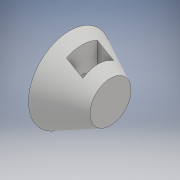
# Autodesk Inventor part: stollen_m4_vierkant
Saved by Autodesk Inventor 2018 (Build 220112000, 112)
## iProperties
Created: 2018-05-14
Part Number: stollen_m4_vierkant
Material: Generic
Document SubType Name: Modeling
Designer: bitbots
Density: 1 g/cm^3
Appearance: Default
Author: bitbots
Autodesk Inventor part; units mm, degrees
ref_plane "XZ Plane" through (0, 0, 0) normal (0, 1, 0) x (-1, 0, 0)
ref_plane "XY Plane" through (0, 0, 0) normal (0, 0, 1) x (1, 0, 0)
ref_plane "Work Plane1" through (7, 0, 0) normal (1, 0, 0) x (0, 1, 0)
sketch "Sketch1" plane through (0, 0, 0) normal (0, 1, 0) x (-1, 0, 0)
  line L0 (0, 0) -> (-10, 0)
  line L1 (0, 0) -> (0, -10)
  line L2 (-10, 0) -> (-10, -5)
  line L3 (-10, -5) -> (0, -10)
  dimension "d0" = 10
  dimension "d1" = 10
  dimension "d2" = 5
  constraints: 8 end point, 2 vertical, 1 horizontal
  measures "d0" distance of L0.start L0.end
  measures "d1" distance of L0.start L1.end
  measures "d2" distance of L0.end L2.end
revolve "Revolution1" add sketch "Sketch1" angle 360 about axis through (0, 0, 0) along (1, 0, 0)
sketch "Sketch2" plane through (7, 0, 0) normal (1, 0, 0) x (0, 1, 0)
  circle A0 centre (0, 0) radius 2.25
  dimension "d5" = 4.5
  constraints: 1 centre point, 1 coincident
  measures "d5" diameter of A0
extrude "Extrusion1" cut sketch "Sketch2" along normal blind 2 and the other way blind 10
sketch "Sketch3" plane through (7, 0, 0) normal (1, 0, 0) x (0, 1, 0)
  line L0 (0, 0) -> (3.75, 0)
  line L1 (3.75, -2.1651) -> (0, -4.3301)
  line L2 (0, -4.3301) -> (-3.75, -2.1651)
  line L3 (-3.75, -2.1651) -> (-3.75, 2.1651)
  line L4 (-3.75, 2.1651) -> (0, 4.3301)
  line L5 (0, 4.3301) -> (3.75, 2.1651)
  line L6 (3.75, 2.1651) -> (3.75, -2.1651)
  line L7 (-3.75, 14.6203) -> (-3.75, 2.1651)
  line L8 (-3.75, 14.6203) -> (3.75, 14.6203)
  line L9 (3.75, 14.6203) -> (3.75, 1.2022)
  line L10 (3.75, 1.2022) -> (-3.75, 1.2022)
  line L11 (-3.75, 1.2022) -> (-3.75, 14.6203)
  dimension "d15" = 3.75
  constraints: 24 end point, 2 horizontal, 2 parallel, 1 coincident, 1 midpoint, 1 perpendicular, 1 point on line, 13 other
  measures "d15" distance of L0.start L0.end
extrude "Extrusion2" cut sketch "Sketch3" against normal blind 4
sketch "Sketch5" plane through (9, 0, 0) normal (-1, 0, 0) x (0, 0, 1)
  circle A0 centre (0, 0) radius 2.25 projected
extrude "Extrusion3" add sketch "Sketch5" along normal up to surface (2 mm away)
body "Solid1"
